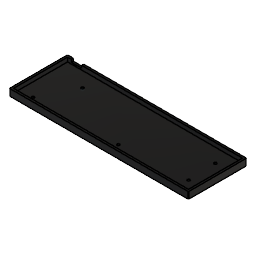
Keyboard Case (Autodesk Fusion 360 design; units mm, degrees)
part number: 2026-01-09-15-44-01-182
Autodesk Fusion 360 part; units mm, degrees
sketch "PCB" plane through (0, 0, 0) normal (0, 0, 1) x (1, 0, 0)
  line L0 (-71.6509, 41.0939) -> (266.3491, 41.0939)
  line L1 (266.3491, 41.0939) -> (266.3491, -61.9061)
  line L2 (266.3491, -61.9061) -> (-71.6509, -61.9061)
  line L3 (-71.6509, -61.9061) -> (-71.6509, 41.0939)
  circle A0 centre (-45.1809, -36.3161) radius 1.6
  circle A1 centre (-14.4909, 13.0239) radius 1.6
  circle A2 centre (115.9291, -47.8061) radius 1.6
  circle A3 centre (243.8291, -38.8761) radius 1.6
  circle A4 centre (241.5491, 15.1939) radius 1.6
  line L4 (-60.6509, 41.0939) -> (-51.6509, 41.0939)
  line L5 (-51.6509, 41.0939) -> (-51.6509, 34)
  line L6 (-51.6509, 34) -> (-60.6509, 34)
  line L7 (-60.6509, 34) -> (-60.6509, 41.0939)
  point P0 (-45.4739, -36.5361)
  point P1 (-40.6298, 20.2839)
  dimension "d1" = 338
  dimension "d2" = 103
  dimension "d3" = 3.2
  dimension "d4" = 25.59
  dimension "d5" = 26.47
  dimension "d6" = 3.2
  dimension "d7" = 28.07
  dimension "d8" = 57.16
  dimension "d9" = 3.2
  dimension "d10" = 14.1
  dimension "d11" = 150.42
  dimension "d12" = 3.2
  dimension "d13" = 22.52
  dimension "d14" = 23.03
  dimension "d15" = 3.2
  dimension "d16" = 24.8
  dimension "d17" = 25.9
  dimension "d32" = 11
  dimension "d33" = 20
  constraint horizontal L0
  constraint vertical L1
  constraint horizontal L2
  constraint vertical L3
  constraint horizontal L4
  constraint vertical L5
  constraint horizontal L6
  constraint vertical L7
  constraint coincident L0 L4.start
  measures "d1" distance of L0.start L0.end
  measures "d2" distance of L0.start L2.end
  measures "d3" diameter of A0
  measures "d4" distance of L2 A0.centre
  measures "d5" distance of L3 A0.centre
  measures "d6" diameter of A1
  measures "d7" distance of L0 A1.centre
  measures "d8" distance of L3 A1.centre
  measures "d9" diameter of A2
  measures "d10" distance of L2 A2.centre
  measures "d11" distance of L1 A2.centre
  measures "d12" diameter of A3
  measures "d13" distance of L1 A3.centre
  measures "d14" distance of L2 A3.centre
  measures "d15" diameter of A4
  measures "d16" distance of L1 A4.centre
  measures "d17" distance of L0 A4.centre
  measures "d32" distance of L3 L7
  measures "d33" distance of L3 L5
sketch "Sketch2" plane through (0, 0, 0) normal (0, 0, 1) x (1, 0, 0)
  line L0 (-76.6509, 46.0939) -> (271.3491, 46.0939)
  line L1 (271.3491, 46.0939) -> (271.3491, -66.9061)
  line L2 (271.3491, -66.9061) -> (-76.6509, -66.9061)
  line L3 (-76.6509, -66.9061) -> (-76.6509, 46.0939)
  line L4 (-71.6509, 41.0939) -> (266.3491, 41.0939)
  line L5 (-71.6509, -61.9061) -> (-71.6509, 41.0939)
  line L6 (266.3491, -61.9061) -> (-71.6509, -61.9061)
  line L7 (266.3491, 41.0939) -> (266.3491, -61.9061)
  line L8 (-72.6509, 42.0939) -> (267.3491, 42.0939)
  line L9 (267.3491, 42.0939) -> (267.3491, -62.9061)
  line L10 (267.3491, -62.9061) -> (-72.6509, -62.9061)
  line L11 (-72.6509, -62.9061) -> (-72.6509, 42.0939)
  line L12 (-51.6509, 46.0939) -> (-51.6509, 39)
  line L13 (-60.6509, 39) -> (-60.6509, 46.0939)
  line L14 (-51.6509, 39) -> (-60.6509, 39)
  dimension "d18" = 5
  dimension "d19" = 5
  dimension "d20" = 5
  dimension "d21" = 5
  dimension "d24" = 4
  dimension "d25" = 4
  dimension "d26" = 4
  dimension "d27" = 4
  constraint horizontal L0
  constraint vertical L1
  constraint horizontal L2
  constraint vertical L3
  constraint horizontal L8
  constraint vertical L9
  constraint horizontal L10
  constraint vertical L11
  constraint vertical L12
  constraint horizontal L14
  constraint vertical L13
  measures "d18" distance of L0 L4
  measures "d19" distance of L3 L5
  measures "d20" distance of L2 L6
  measures "d21" distance of L1 L7
  measures "d24" distance of L2 L10
  measures "d25" distance of L0 L8
  measures "d26" distance of L3 L11
  measures "d27" distance of L1 L9
extrude "Extrude1" add sketch "Sketch2" along normal blind 5 contours L4 L5 L6 L7 L12 L13 L14 | L4 L12 L13 L14
extrude "Extrude2" add sketch "Sketch2" along normal blind 5 contours L4 L5 L6 L7 L8 L9 L10 L11 L12 L13 | L4 L8 L12 L13
extrude "Extrude3" add sketch "Sketch2" along normal blind 13 contours L0 L1 L2 L3 L8 L9 L10 L11 L12 L13 | L0 L8 L12 L13
sketch "Sketch3" plane through (0, 0, 13) normal (0, 0, 1) x (-1, 0, 0)
  line L0 (-267.3491, 62.9061) -> (72.6509, 62.9061)
  line L1 (72.6509, 62.9061) -> (72.6509, -42.0939)
  line L2 (72.6509, -42.0939) -> (-267.3491, -42.0939)
  line L3 (-267.3491, -42.0939) -> (-267.3491, 62.9061)
  line L4 (76.6509, 66.9061) -> (-271.3491, 66.9061)
  line L5 (-271.3491, 66.9061) -> (-271.3491, -46.0939)
  line L6 (-271.3491, -46.0939) -> (76.6509, -46.0939)
  line L7 (76.6509, -46.0939) -> (76.6509, 66.9061)
  line L8 (65.1904, -46.0939) -> (45.472, -46.0939)
  line L9 (45.472, -46.0939) -> (45.472, -42.0939)
  line L10 (45.472, -42.0939) -> (65.1904, -42.0939)
  line L11 (65.1904, -42.0939) -> (65.1904, -46.0939)
  constraint horizontal L8
  constraint vertical L9
  constraint horizontal L10
  constraint vertical L11
  constraint coincident L2 L9.end
  constraint coincident L6 L8.start
extrude "Extrude4" cut sketch "Sketch3" against normal blind 5 contours L2 L6 L8 L9 L10 L11
sketch "HOLWS" plane through (0, 0, 5) normal (0, 0, 1) x (-1, 0, 0)
  line L0 (72.6509, 62.9061) -> (-267.3491, 62.9061)
  line L1 (-267.3491, 62.9061) -> (-267.3491, -42.0939)
  line L2 (-267.3491, -42.0939) -> (72.6509, -42.0939)
  line L3 (72.6509, -42.0939) -> (72.6509, 62.9061)
  circle A0 centre (14.5, -13) radius 2.15
  circle A1 centre (46.6409, 51.0461) radius 2.15
  circle A2 centre (-115.929, 47.8061) radius 2.15
  circle A3 centre (-243.8291, 38.876) radius 2.15
  circle A4 centre (-241.5493, -15.1935) radius 2.15
  dimension "d48" = 4.3
  dimension "d49" = 4.3
  dimension "d50" = 4.3
  dimension "d51" = 4.3
  dimension "d52" = 4.3
  dimension "d57" = 26.01
  dimension "d58" = 11.86
  measures "d48" diameter of A0
  measures "d49" diameter of A1
  measures "d50" diameter of A2
  measures "d51" diameter of A3
  measures "d52" diameter of A4
  measures "d57" distance of L3 A1.centre
  measures "d58" distance of L0 A1.centre
fillet "Fillet1" radius 1 1 edges at (-76.6509, -66.9061, 6.5)
fillet "Fillet2" radius 1 1 edges at (-76.6509, 46.0939, 6.5)
fillet "Fillet3" radius 1 1 edges at (271.3491, -66.9061, 6.5)
fillet "Fillet4" radius 1 1 edges at (271.3491, 46.0939, 6.5)
sketch "Sketch5" plane through (0, 0, 0) normal (0, 0, 1) x (1, 0, 0)
  line L0 (256.3491, 36.2293) -> (-61.6509, 36.2293)
  line L1 (-61.6509, 36.2293) -> (-61.6509, 24.2668)
  line L2 (-61.6509, 24.2668) -> (256.3491, 24.2668)
  line L3 (256.3491, 24.2668) -> (256.3491, 36.2293)
  line L4 (-71.6509, -61.9061) -> (-71.6509, 41.0939)
  line L5 (266.3491, 41.0939) -> (266.3491, -61.9061)
  dimension "d44" = 10
  dimension "d45" = 10
  constraint horizontal L0
  constraint vertical L1
  constraint horizontal L2
  constraint vertical L3
  measures "d44" distance of L1 L4
  measures "d45" distance of L3 L5
extrude "Extrude5" add sketch "Sketch5" against normal blind 3
extrude "Extrude6" cut sketch "HOLWS" against normal blind 3.2 contours A0 | A1 | A2 | A3 | A4
chamfer "Chamfer1" distance 0.35 angle 45 1 edges at (-12.4955, 12.2225, 5)
chamfer "Chamfer2" distance 0.35 angle 45 4 edges at (-44.6364, -51.8236, 5) (117.9335, -48.5836, 5) (243.5538, 14.416, 5) (245.8336, -39.6534, 5)
move_body "Move1" bodies 1 to x (1, 0, 0) y (0, 1, 0) z (0, 0, 1) at (60, 0, 0)
move_body "Move2" bodies 1 to x (1, 0, 0) y (0, 1, 0) z (0, 0, 1) at (0, -5, 0)
move_body "Move3" bodies 1 to x (1, 0, 0) y (0, 1, 0) z (0, 0, 1) at (-60, 5, 0)
sketch "Sketch6" plane through (0, 0, 1.8) normal (0, 0, 1) x (-1, 0, 0)
  circle A0 centre (14.5, -13) radius 2.15
